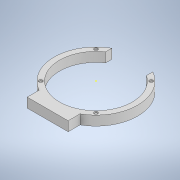
# Autodesk Inventor part: expo5
Saved by Autodesk Inventor 2020 (Build 240168000, 168)
## iProperties
Created: 2020-02-19
Part Number: expo5
Material: Generic
Document SubType Name: Modeling
Designer: Aryan
Density: 1 g/cm^3
Appearance: Default
Author: Aryan
Autodesk Inventor part; units mm, degrees
ref_plane "YZ Plane" through (0, 0, 0) normal (1, 0, 0) x (0, 1, 0)
ref_plane "XZ Plane" through (0, 0, 0) normal (0, 1, 0) x (-1, 0, 0)
ref_plane "XY Plane" through (0, 0, 0) normal (0, 0, 1) x (1, 0, 0)
sketch "Sketch1" plane through (0, 0, 0) normal (0, 1, 0) x (-1, 0, 0)
  circle A0 centre (0, 0) radius 35
  dimension "d0" = 70
  constraints: 1 centre point, 1 coincident
  measures "d0" diameter of A0
extrude "Extrusion1" add sketch "Sketch1" along normal blind 8
sketch "Sketch2" plane through (0, 8, 0) normal (0, 1, 0) x (1, 0, 0)
  circle A0 centre (0, 0) radius 30.5
  dimension "d3" = 61
  constraints: 1 centre point, 1 coincident
  measures "d3" diameter of A0
extrude "Extrusion2" cut sketch "Sketch2" against normal blind 8
sketch "Sketch3" plane through (0, 8, 0) normal (0, 1, 0) x (1, 0, 0)
  circle A0 centre (0, 0) radius 30.5 projected
  line L0 (0, -30.5) -> (-17.1683, -30.5)
  circle A1 centre (0, 0) radius 35 projected
  line L1 (-17.1683, -30.5) -> (17.1677, -30.5)
  line L2 (17.1677, -30.5) -> (17.1677, -40.5)
  line L3 (17.1677, -40.5) -> (-17.1683, -40.5)
  line L4 (-17.1683, -40.5) -> (-17.1683, -30.5)
  dimension "d6" = 34.336
  dimension "d7" = 10
  constraints: 10 end point, 2 horizontal, 2 parallel, 1 perpendicular, 1 vertical alignment, 3 other
  measures "d6" distance of L2.end L3.end
  measures "d7" distance of L1.end L2.end
extrude "Extrusion3" add sketch "Sketch3" against normal blind 8 contours L1 A1 L0 | A1 L2 L3 L4 picked at (9.255, -31.4525)
sketch "Sketch4" plane through (0, 8, 0) normal (0, 1, 0) x (1, 0, 0)
  line L0 (-17.1683, -40.5) -> (-17.1683, -30.5) projected
  line L1 (-17.1683, -30.5) -> (-17.1683, 30.5)
  arc A0 (17.1677, -30.5003) -> (-17.1683, -30.5) centre (0, 0) ccw projected
  line L2 (17.1677, -30.5003) -> (17.1677, 30.5)
  circle A1 centre (0, 0) radius 30.5 projected
  line L3 (-17.1683, 25.2091) -> (17.1677, 25.2091)
  line L4 (17.1677, 25.2091) -> (17.1677, 37.2402)
  line L5 (17.1677, 37.2402) -> (-17.1683, 37.2402)
  line L6 (-17.1683, 37.2402) -> (-17.1683, 25.2091)
  point P0 (17.1677, 30.5)
  constraints: 12 end point, 2 parallel, 2 vertical, 1 horizontal, 1 perpendicular, 1 point on circle, 1 point on line, 2 other
extrude "Extrusion4" cut sketch "Sketch4" against normal blind 8 contours L1 A0 L2 A1 | A1 L3 | L6 L5 L4 A0
sketch "Sketch5" plane through (0, 8, 0) normal (0, 1, 0) x (1, 0, 0)
  point P0 (0, 0)
sketch "Sketch6" plane through (0, 8, 0) normal (0, 1, 0) x (1, 0, 0)
  line L0 (0, 0) -> (-23.1577, 23.1577)
  line L1 (0, 0) -> (32.75, 0) construction
  circle A0 centre (-23.1577, 23.1577) radius 1.5
  dimension "d12" = 32.75
  dimension "d13" = 135
  dimension "d14" = 3
  constraints: 4 end point, 1 centre point, 1 coincident, 1 equal length, 1 horizontal
  measures "d12" distance of L0.start L0.end
  measures "d13" angle of L1 L0
  measures "d14" diameter of A0
extrude "Extrusion5" cut sketch "Sketch6" against normal blind 1
sketch "Sketch7" plane through (0, 8, 0) normal (0, 1, 0) x (1, 0, 0)
  line L0 (0, 0) -> (-23.1577, -23.1577)
  line L1 (0, 0) -> (32.75, 0) construction
  circle A0 centre (-23.1577, -23.1577) radius 1.5
  dimension "d17" = 32.75
  dimension "d18" = 135
  dimension "d19" = 3
  constraints: 4 end point, 1 centre point, 1 coincident, 1 equal length, 1 horizontal
  measures "d17" distance of L0.start L0.end
  measures "d18" angle of L0 L1
  measures "d19" diameter of A0
extrude "Extrusion6" cut sketch "Sketch7" against normal blind 1
sketch "Sketch8" plane through (0, 8, 0) normal (0, 1, 0) x (1, 0, 0)
  line L0 (0, 0) -> (23.1577, -23.1577)
  line L1 (0, 0) -> (32.75, 0) construction
  circle A0 centre (23.1577, -23.1577) radius 1.5
  dimension "d22" = 32.75
  dimension "d23" = 45
  dimension "d24" = 3
  constraints: 4 end point, 1 centre point, 1 coincident, 1 equal length, 1 horizontal
  measures "d22" distance of L0.start L0.end
  measures "d23" angle of L0 L1
  measures "d24" diameter of A0
extrude "Extrusion7" cut sketch "Sketch8" against normal blind 1
sketch "Sketch9" plane through (0, 8, 0) normal (0, 1, 0) x (1, 0, 0)
  line L0 (0, 0) -> (23.1577, 23.1577)
  line L1 (0, 0) -> (32.75, 0) construction
  circle A0 centre (23.1577, 23.1577) radius 1.5
  dimension "d27" = 32.75
  dimension "d28" = 45
  dimension "d29" = 3
  constraints: 4 end point, 1 centre point, 1 coincident, 1 equal length, 1 horizontal
  measures "d27" distance of L0.start L0.end
  measures "d28" angle of L1 L0
  measures "d29" diameter of A0
extrude "Extrusion8" cut sketch "Sketch9" against normal blind 1
sketch "Sketch10" plane through (0, 8, 0) normal (0, 1, 0) x (1, 0, 0)
  point P0 (0, 0)
body "Solid1"
